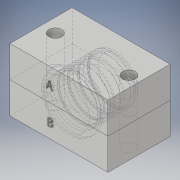
# Autodesk Inventor part: 7_8-Cap
Saved by Autodesk Inventor 2019.3 (Build 233278000, 278)
## iProperties
Created: 2018-12-29
Part Number: 7_8-Cap
Material: Generic
Document SubType Name: Modeling
Designer: eroldan
Density: 1 g/cm^3
Appearance: Default
Author: eroldan
Autodesk Inventor part; units mm, degrees
ref_plane "YZ Plane" through (0, 0, 0) normal (1, 0, 0) x (0, 1, 0)
ref_plane "XZ Plane" through (0, 0, 0) normal (0, 1, 0) x (-1, 0, 0)
ref_plane "XY Plane" through (0, 0, 0) normal (0, 0, 1) x (1, 0, 0)
sketch "Sketch1" plane through (0, 0, 0) normal (0, 0, 1) x (1, 0, 0)
  circle A0 centre (0, 0) radius 11.1125
  circle A1 centre (0, 0) radius 9.5
  dimension "d0" = 22.225
  dimension "d1" = 19
  constraints: 2 centre point, 2 coincident
  measures "d0" diameter of A0
  measures "d1" diameter of A1
extrude "Extrusion1" add sketch "Sketch1" against normal blind 3
extrude "Extrusion2" add sketch "Sketch1" against normal blind 20 contours A1
sketch "Sketch2" plane through (0, 0, 0) normal (0, 1, 0) x (-1, 0, 0)
  line L0 (9.5, -4.1691) -> (7.5, -5.8103)
  line L1 (7.5, -5.8103) -> (9.5, -5.8103)
  line L2 (0, -24) -> (0, 4) projected
  line L3 (9.5, -3) -> (9.5, -20) projected
  point P0 (0, 0)
  dimension "d9" = 2
  constraints: 4 end point, 2 point on line, 1 perpendicular
  measures "d9" distance of L0.end L1.end
revolve "Revolution2" cut sketch "Sketch2" angle 360 about axis through (0, 0, -10) along (0, 0, 1)
fillet "Fillet1" radius 0.5 1 edges at (7.5, 0, -5.8103)
pattern_linear "Rectangular Pattern1" count 4 spacing 4 along (0, 0, -1) of "Revolution2", "Fillet1"
fillet "Fillet2" radius 2 2 edges at (-11.1125, 0, 0) (-9.5, 0, -20)
sketch "Sketch3" plane through (0, 0, 0) normal (0, 1, 0) x (-1, 0, 0)
  line L0 (20.0537, -22.2142) -> (-19.0305, -22.2142)
  line L1 (-19.0305, -22.2142) -> (-19.0305, 2.5379)
  line L2 (-19.0305, 2.5379) -> (20.0537, 2.5379)
  line L3 (20.0537, 2.5379) -> (20.0537, -22.2142)
  point P0 (0, 0)
  constraints: 8 end point, 2 parallel, 1 horizontal, 1 perpendicular
extrude "Extrusion3" add sketch "Sketch3" along normal mid plane 25 separate body
sketch "Sketch6" plane through (-20.0537, 12.5, 2.5379) normal (0, 0, 1) x (1, 0, 0)
  line L0 (14.4727, -5.0136) -> (17.0267, -5.0136) construction
  line L1 (17.0267, -5.0136) -> (17.0267, -8.0616) construction
  line L2 (17.0267, -8.0616) -> (14.4727, -8.0616) construction
  line L3 (14.4727, -8.0616) -> (14.4727, -5.0136) construction
  line L4 (14.8054, -17.8569) -> (17.2754, -17.8569) construction
  line L5 (17.2754, -17.8569) -> (17.2754, -20.9049) construction
  line L6 (17.2754, -20.9049) -> (14.8054, -20.9049) construction
  line L7 (14.8054, -20.9049) -> (14.8054, -17.8569) construction
  line L8 (14.4529, -8.0616) -> (15.4805, -5.0136)
  line L9 (15.4805, -5.0136) -> (15.9794, -5.0136)
  line L10 (15.9794, -5.0136) -> (17.0069, -8.0616)
  line L11 (17.0069, -8.0616) -> (16.5796, -8.0616)
  line L12 (16.5796, -8.0616) -> (16.303, -7.2095)
  line L13 (16.303, -7.2095) -> (15.1396, -7.2095)
  line L14 (15.1396, -7.2095) -> (14.863, -8.0616)
  line L15 (14.863, -8.0616) -> (14.4529, -8.0616)
  line L16 (16.1918, -6.8637) -> (15.7201, -5.4286)
  line L17 (15.7201, -5.4286) -> (15.2508, -6.8637)
  line L18 (15.2508, -6.8637) -> (16.1918, -6.8637)
  spline S0 degree 2 poles (17.1816, -19.9688) (17.1816, -20.196) (17.0087, -20.5443) (16.8654, -20.6579) knots 0 0 0 1 2 2 2
  spline S1 degree 2 poles (16.8654, -20.6579) (16.6925, -20.7913) (16.2998, -20.9049) (15.9886, -20.9049) knots 0 0 0 1 2 2 2
  line L19 (15.9886, -20.9049) -> (15.1142, -20.9049)
  line L20 (15.1142, -20.9049) -> (15.1142, -17.8569)
  line L21 (15.1142, -17.8569) -> (15.9219, -17.8569)
  spline S2 degree 2 poles (15.9219, -17.8569) (16.2479, -17.8569) (16.574, -17.8989) (16.7222, -17.9804) knots 0 0 0 1 2 2 2
  spline S3 degree 2 poles (16.7222, -17.9804) (16.8877, -18.0669) (17.0383, -18.3509) (17.0383, -18.5436) knots 0 0 0 1 2 2 2
  spline S4 degree 2 poles (17.0383, -18.5436) (17.0383, -18.7585) (16.8111, -19.0993) (16.611, -19.1957) knots 0 0 0 1 2 2 2
  line L22 (16.611, -19.1957) -> (16.611, -19.2105)
  spline S5 degree 2 poles (16.611, -19.2105) (16.8827, -19.2846) (17.1816, -19.6773) (17.1816, -19.9688) knots 0 0 0 1 2 2 2
  spline S6 degree 2 poles (16.7592, -19.9861) (16.7592, -19.8132) (16.6604, -19.5909) (16.5122, -19.5118) knots 0 0 0 1 2 2 2
  spline S7 degree 2 poles (16.5122, -19.5118) (16.4159, -19.4624) (16.1886, -19.4328) (15.9787, -19.4328) knots 0 0 0 1 2 2 2
  line L23 (15.9787, -19.4328) -> (15.5193, -19.4328)
  line L24 (15.5193, -19.4328) -> (15.5193, -20.5591)
  line L25 (15.5193, -20.5591) -> (15.8478, -20.5591)
  spline S8 degree 2 poles (15.8478, -20.5591) (16.1145, -20.5591) (16.4208, -20.5097) (16.5394, -20.4307) knots 0 0 0 1 2 2 2
  spline S9 degree 2 poles (16.5394, -20.4307) (16.653, -20.3492) (16.7592, -20.1466) (16.7592, -19.9861) knots 0 0 0 1 2 2 2
  spline S10 degree 2 poles (16.616, -18.6004) (16.616, -18.4917) (16.5419, -18.3287) (16.4603, -18.2818) knots 0 0 0 1 2 2 2
  spline S11 degree 2 poles (16.4603, -18.2818) (16.3615, -18.2274) (16.1219, -18.2027) (15.9071, -18.2027) knots 0 0 0 1 2 2 2
  line L26 (15.9071, -18.2027) -> (15.5193, -18.2027)
  line L27 (15.5193, -18.2027) -> (15.5193, -19.0944)
  line L28 (15.5193, -19.0944) -> (15.9787, -19.0944)
  spline S12 degree 2 poles (15.9787, -19.0944) (16.1689, -19.0944) (16.3492, -19.0549) (16.4455, -18.9931) knots 0 0 0 1 2 2 2
  spline S13 degree 2 poles (16.4455, -18.9931) (16.5394, -18.9338) (16.616, -18.7436) (16.616, -18.6004) knots 0 0 0 1 2 2 2
  point P0 (20.0537, -12.5)
  constraints: 4 other
emboss "Emboss1" sketch "Sketch6" operation cut depth 0.5 direction (0, 0, -1)
sketch "Sketch4" plane through (0, 12.5, 0) normal (0, 1, 0) x (1, 0, 0)
  point P0 (0, 0)
  point P1 (14.6637, 10.1998)
  point P2 (-14.5571, 10.0589)
hole "Hole1" at (14.6637, 12.5, -10.1998) at (-14.5571, 12.5, -10.0589) direction (0, -1, 0) diameter 5.1 end through all both bodies 2
combine bodies "Combine1" operation type subtract main body 2 bodies to subtract 1
split body "Split1" result two bodies by plane through (0, 0, 0) normal (0, 1, 0) bodies 2 first body at (-4.6298, 12, -1.0248)
